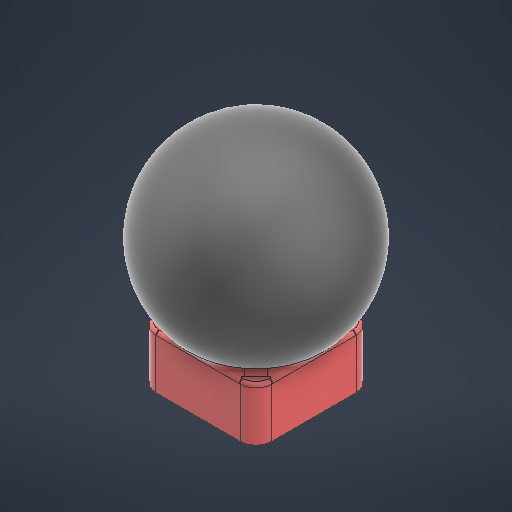
# Autodesk Inventor part: foot
Saved by Autodesk Inventor 2027 (Build 310192060, 192F)
## iProperties
Created: 2026-08-17
Part Number: foot
Material: Ogólny
Document SubType Name: Modeling
Designer: User
Density: 1 g/cm^3
Appearance: Domyślna
Author: User
Autodesk Inventor part; units mm, degrees
ref_plane "YZ Plane" through (0, 0, 0) normal (1, 0, 0) x (0, 1, 0)
ref_plane "XZ Plane" through (0, 0, 0) normal (0, 1, 0) x (-1, 0, 0)
sketch "Szkic1" plane through (0, 0, 0) normal (0, 1, 0) x (-1, 0, 0)
  circle A0 centre (0, 0) radius 5
  line L0 (-5.7037, -5.5) -> (5.2963, -5.5)
  line L1 (5.2963, -5.5) -> (5.2963, 5.5)
  line L2 (5.2963, 5.5) -> (-5.7037, 5.5)
  line L3 (-5.7037, 5.5) -> (-5.7037, -5.5)
  line L4 (-5.7037, -5.5) -> (5.2963, 5.5) construction
  line L5 (5.2963, -5.5) -> (-5.7037, 5.5) construction
  point P0 (-0.2037, 0)
  dimension "d0" = 10
  dimension "d1" = 11
  dimension "d2" = 11
  constraints: 12 end point, 2 midpoint, 2 parallel, 1 centre point, 1 coincident, 1 horizontal, 1 perpendicular
  measures "d0" diameter of A0
  measures "d1" distance of L2.end L1.end
  measures "d2" distance of L1.end L0.end
extrude "Wyciągnięcie proste1" add sketch "Szkic1" along normal blind 5
ref_plane "Płaszczyzna konstrukcyjna1" through (-5.2963, 0, 0) normal (0, 0, 1) x (1, 0, 0)
sketch "Szkic2" plane through (-5.2963, 0, 0) normal (0, 0, 1) x (1, 0, 0)
  line L0 (0, 5) -> (11, 5) projected
  line L1 (0, 5) -> (11, 5)
  line L2 (5.5, 5) -> (5.5, 12)
  line L3 (5.5, 5) -> (12.5, 5) construction
  line L4 (11, 0) -> (11, 5) projected
  circle A0 centre (5.5, 12) radius 8.9022
  line L5 (5.5, 12) -> (5.5, 20.9022)
  line L6 (5.5, 5) -> (5.5, 3.0978)
  point P0 (5.2963, 0)
  dimension "d6" = 7
  dimension "d7" = 90
  constraints: 10 end point, 3 point on circle, 3 vertical, 2 horizontal, 1 centre point, 1 coincident, 1 midpoint, 1 perpendicular
  measures "d6" distance of L2.start L2.end
  measures "d7" angle of L3 L2
revolve "Obrót1" add sketch "Szkic2" angle 360 about axis through (0.2037, 5, 0) along (0, 1, 0) picked at (7.3333, 7.3333) contours L2 L5 A0 L0
fillet "Zaokrąglenie2" radius 0.3 12 edges at (-3.6854, 5, 3.8891) (-5.2963, 5, 2.75) (-2.5463, 5, 5.5) (-3.6854, 5, -3.8891) (-2.5463, 5, -5.5) (-5.2963, 5, -2.75) (4.0928, 5, -3.8891) (2.9537, 5, -5.5) (5.7037, 5, -2.75) (4.0928, 5, 3.8891) (5.7037, 5, 2.75) (2.9537, 5, 5.5)
fillet "Zaokrąglenie3" radius 1.5 8 edges at (-5.2084, 4.9121, 5.4121) (-5.2963, 2.35, 5.5) (5.6158, 4.9121, 5.4121) (5.7037, 2.35, 5.5) (5.6158, 4.9121, -5.4121) (5.7037, 2.35, -5.5) (-5.2084, 4.9121, -5.4121) (-5.2963, 2.35, -5.5)
